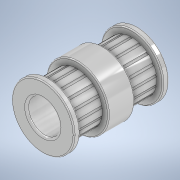
# Autodesk Inventor part: double-head pulley
Saved by Autodesk Inventor 2020.4 (Build 244396000, 396)
## iProperties
Created: 2021-02-19
Part Number: double-head pulley
Material: Aluminum 6061
Document SubType Name: Modeling
Designer: AOB
Mass: 6.07158 g
Surface Area: 23.4663 cm^2
Volume: 2.24873 cm^3
Density: 2.7 g/cm^3
Appearance: Aluminum - Polished
Author: AOB
Autodesk Inventor part; units mm, degrees
ref_plane "YZ Plane" through (0, 0, 0) normal (1, 0, 0) x (0, 1, 0)
ref_plane "XZ Plane" through (0, 0, 0) normal (0, 1, 0) x (-1, 0, 0)
ref_plane "XY Plane" through (0, 0, 0) normal (0, 0, 1) x (1, 0, 0)
sketch "Sketch1" plane through (0, 0, 0) normal (0, 0, 1) x (1, 0, 0)
  circle A0 centre (0, 0) radius 7.735
  arc A1 (-0.2774, 6.2088) -> (0.2774, 6.2088) centre (0, 6.215) ccw
  arc A2 (1.8628, 5.9293) -> (2.3842, 5.7395) centre (2.1257, 5.8402) ccw
  arc A3 (3.7784, 4.9345) -> (4.2035, 4.5779) centre (3.9949, 4.761) ccw
  arc A4 (5.2383, 3.3447) -> (5.5157, 2.8641) centre (5.3823, 3.1075) ccw
  arc A5 (6.0663, 1.3514) -> (6.1627, 0.8049) centre (6.1206, 1.0792) ccw
  arc A6 (6.1627, -0.8049) -> (6.0663, -1.3514) centre (6.1206, -1.0792) ccw
  arc A7 (5.5157, -2.8641) -> (5.2383, -3.3447) centre (5.3823, -3.1075) ccw
  arc A8 (4.2035, -4.5779) -> (3.7784, -4.9345) centre (3.9949, -4.761) ccw
  arc A9 (2.3842, -5.7395) -> (1.8628, -5.9293) centre (2.1257, -5.8402) ccw
  arc A10 (0.2774, -6.2088) -> (-0.2774, -6.2088) centre (0, -6.215) ccw
  arc A11 (-1.8628, -5.9293) -> (-2.3842, -5.7395) centre (-2.1257, -5.8402) ccw
  arc A12 (-3.7784, -4.9345) -> (-4.2035, -4.5779) centre (-3.9949, -4.761) ccw
  arc A13 (-5.2383, -3.3447) -> (-5.5157, -2.8641) centre (-5.3823, -3.1075) ccw
  arc A14 (-6.0663, -1.3514) -> (-6.1627, -0.8049) centre (-6.1206, -1.0792) ccw
  arc A15 (-6.1627, 0.8049) -> (-6.0663, 1.3514) centre (-6.1206, 1.0792) ccw
  arc A16 (-5.5157, 2.8641) -> (-5.2383, 3.3447) centre (-5.3823, 3.1075) ccw
  arc A17 (-4.2035, 4.5779) -> (-3.7784, 4.9345) centre (-3.9949, 4.761) ccw
  arc A18 (-2.3842, 5.7395) -> (-1.8628, 5.9293) centre (-2.1257, 5.8402) ccw
  arc A19 (-0.2774, 6.2088) -> (-1.8628, 5.9293) centre (0, 0) ccw
  arc A20 (-2.3842, 5.7395) -> (-3.7784, 4.9345) centre (0, 0) ccw
  arc A21 (-4.2035, 4.5779) -> (-5.2383, 3.3447) centre (0, 0) ccw
  arc A22 (-5.5157, 2.8641) -> (-6.0663, 1.3514) centre (0, 0) ccw
  arc A23 (3.7784, 4.9345) -> (2.3842, 5.7395) centre (0, 0) ccw
  arc A24 (1.8628, 5.9293) -> (0.2774, 6.2088) centre (0, 0) ccw
  arc A25 (5.2383, 3.3447) -> (4.2035, 4.5779) centre (0, 0) ccw
  arc A26 (6.0663, 1.3514) -> (5.5157, 2.8641) centre (0, 0) ccw
  arc A27 (6.1627, -0.8049) -> (6.1627, 0.8049) centre (0, 0) ccw
  arc A28 (5.5157, -2.8641) -> (6.0663, -1.3514) centre (0, 0) ccw
  arc A29 (4.2035, -4.5779) -> (5.2383, -3.3447) centre (0, 0) ccw
  arc A30 (2.3842, -5.7395) -> (3.7784, -4.9345) centre (0, 0) ccw
  arc A31 (0.2774, -6.2088) -> (1.8628, -5.9293) centre (0, 0) ccw
  arc A32 (-1.8628, -5.9293) -> (-0.2774, -6.2088) centre (0, 0) ccw
  arc A33 (-3.7784, -4.9345) -> (-2.3842, -5.7395) centre (0, 0) ccw
  arc A34 (-5.2383, -3.3447) -> (-4.2035, -4.5779) centre (0, 0) ccw
  arc A35 (-6.1627, 0.8049) -> (-6.1627, -0.8049) centre (0, 0) ccw
  arc A36 (-6.0663, -1.3514) -> (-5.5157, -2.8641) centre (0, 0) ccw
  circle A37 centre (0, 0) radius 6.215
  point P0 (-6.0663, -1.3514)
  point P1 (-6.1627, -0.8049)
  point P2 (-6.1627, 0.8049)
  point P3 (-6.0663, 1.3514)
  point P4 (-3.7784, 4.9345)
  point P5 (-2.3842, 5.7395)
  point P6 (-1.8628, 5.9293)
  point P7 (0.2774, 6.2088)
  point P8 (1.8628, 5.9293)
  point P9 (2.3842, 5.7395)
  point P10 (5.5157, 2.8641)
  point P11 (6.0663, 1.3514)
  point P12 (6.1627, -0.8049)
  point P13 (5.2383, -3.3447)
  point P14 (1.8628, -5.9293)
  point P15 (0.2774, -6.2088)
  point P16 (-0.2774, -6.2088)
  point P17 (-1.8628, -5.9293)
  point P18 (-2.3842, -5.7395)
  point P19 (-5.5157, -2.8641)
  dimension "d0" = 15.47
  dimension "d2" = 0.555
  dimension "d5" = 360
  constraints: 72 point on circle, 37 centre point, 3 coincident, 76 other
  measures "d0" diameter of A0
  measures "d2" diameter of A1
extrude "Extrusion1" add sketch "Sketch1" along normal mid plane 20.5 contours A1 A24 A2 A23 A3 A25 A4 A26 A5 A27 A6 A28 A7 A29 A8 A30 A9 A31 A10 A32 A11 A33 A12 A34 A13 A36 A14 A35 A15 A22 A16 A21 A17 A20 A18 A19
extrude "Extrusion2" add sketch "Sketch1" along normal mid plane 6.5
sketch "Sketch2" plane through (0, 0, 10.25) normal (0, 0, 1) x (1, 0, 0)
  arc A0 (6.1627, -0.8049) -> (6.1627, 0.8049) centre (0, 0) ccw projected
  circle A1 centre (0, 0) radius 7.735
  constraints: 1 centre point, 1 coincident
extrude "Extrusion3" add sketch "Sketch2" along normal blind 1.5
sketch "Sketch3" plane through (0, 0, -10.25) normal (0, 0, -1) x (-1, 0, 0)
  circle A0 centre (0, 0) radius 7.735
  constraints: 1 centre point, 1 coincident
extrude "Extrusion4" add sketch "Sketch3" along normal blind 1.5
hole "Hole1" at (0, 0, 10.25) direction (0, 0, -1) diameter 8 end through all both
fillet "Fillet1" radius 0.5 1 edges at (0, 4, -11.75) inverted yes
fillet "Fillet2" radius 0.5 1 edges at (0, 4, 11.75)
fillet "Fillet3" radius 0.25 1 edges at (-7.735, 0, 11.75) curvature continuous yes
fillet "Fillet4" radius 0.25 1 edges at (-7.735, 0, 10.25)
fillet "Fillet5" radius 0.25 2 edges at (7.735, 0, -11.75) (7.735, 0, -10.25)
fillet "Fillet6" radius 0.25 2 edges at (-7.735, 0, 3.25) (-7.735, 0, -3.25)
body "Solid1"
